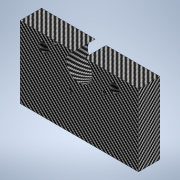
# Autodesk Inventor part: Placa6 Base1
Saved by Autodesk Inventor 2022 (Build 260153000, 153)
## iProperties
Created: 2021-11-08
Part Number: Placa6 Base1
Material: CFRP
Document SubType Name: Modeling
Designer: Samuel Gómez
Density: 1.43 g/cm^3
Appearance: Carbon Fiber
Author: Samuel Gómez
Autodesk Inventor part; units mm, degrees
ref_plane "YZ Plane" through (0, 0, 0) normal (1, 0, 0) x (0, 1, 0)
ref_plane "XZ Plane" through (0, 0, 0) normal (0, 1, 0) x (-1, 0, 0)
ref_plane "XY Plane" through (0, 0, 0) normal (0, 0, 1) x (1, 0, 0)
sketch "Boceto1" plane through (0, 0, 0) normal (0, 0, 1) x (1, 0, 0)
  line L0 (0, 0) -> (100, 0)
  line L1 (100, 0) -> (100, 61)
  line L2 (100, 61) -> (0, 61)
  line L3 (0, 61) -> (0, 0)
  dimension "d0" = 61
  dimension "d1" = 100
  constraints: 8 end point, 2 parallel, 1 horizontal, 1 perpendicular
  measures "d0" distance of L2.end L0.start
  measures "d1" distance of L0.start L0.end
extrude "Extrusión1" add sketch "Boceto1" along normal blind 18
sketch "Boceto2" plane through (0, 0, 18) normal (0, 0, 1) x (1, 0, 0)
  circle A0 centre (50, 51) radius 11
  line L0 (0, 61) -> (0, 0) projected
  line L1 (100, 61) -> (0, 61) projected
  line L2 (50, 51) -> (20, 51) construction
  circle A1 centre (20, 51) radius 4
  line L3 (50, 51) -> (50, 22.8333) construction
  circle A2 centre (80, 51) radius 4
  circle A3 centre (29.6074, 59.04) radius 1.5
  line L4 (29.6074, 59.04) -> (50, 51) construction
  line L5 (50, 51) -> (78.7272, 39.674) construction
  circle A4 centre (70.3926, 42.96) radius 1.5
  line L6 (50, 51) -> (39.3624, 24.0188) construction
  circle A5 centre (41.96, 30.6074) radius 1.5
  line L7 (50, 51) -> (25.0918, 40.1786)
  line L8 (50, 51) -> (59.4119, 29.3362)
  point P0 (54.5826, 61)
  point P1 (45.4174, 61)
  dimension "d4" = 22
  dimension "d5" = 50
  dimension "d6" = 10
  dimension "d7" = 8
  dimension "d8" = 30
  dimension "d9" = 3
  dimension "d10" = 1.96
  dimension "d12" = 3
  dimension "d13" = 90
  dimension "d14" = 3
  dimension "d17" = 45
  dimension "d18" = 15.5
  dimension "d19" = 15.5
  dimension "d20" = 45
  dimension "d21" = 15.5
  constraints: 14 end point, 6 centre point, 2 coincident, 2 point on line, 1 collinear, 1 horizontal, 1 symmetric about line, 1 vertical, 1 other
  measures "d4" diameter of A0
  measures "d5" distance from line of L0 L2.start
  measures "d6" distance from line of L2.start L1
  measures "d7" diameter of A1
  measures "d8" distance of L2.start A1.centre
  measures "d9" diameter of A3
  measures "d10" distance from line of L1 L4.start
  measures "d12" diameter of A4
  measures "d13" angle of L6 L4
  measures "d14" diameter of A5
  measures "d17" angle of L7 L4
  measures "d18" distance from line of L7 L4.start
  measures "d19" distance from line of L7 A5.centre
  measures "d20" angle of L8 L5
  measures "d21" distance from line of L8 A4.centre
extrude "Extrusión2" cut sketch "Boceto2" against normal blind 18 contours A0 L8 L7 L1 | A0 L7 L8 | A1 | A2 | A3 | A4 | A5
